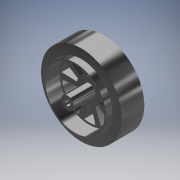
# Autodesk Inventor part: Wheel for rc car
Saved by Autodesk Inventor 2019 (Build 230136000, 136)
## iProperties
Created: 2020-03-11
Part Number: Wheel for rc car
Material: Generic
Document SubType Name: Modeling
Designer: 108863
Density: 1 g/cm^3
Appearance: Knurled 45
Author: 108863
Autodesk Inventor part; units mm, degrees
ref_plane "YZ Plane" through (0, 0, 0) normal (1, 0, 0) x (0, 1, 0)
ref_plane "XZ Plane" through (0, 0, 0) normal (0, 1, 0) x (-1, 0, 0)
sketch "Sketch2" plane through (0, 0, 0) normal (0, 0, 1) x (1, 0, 0)
  circle A0 centre (0, 0) radius 10.9728
  dimension "d5" = 21.9456
  constraints: 1 centre point, 1 coincident
  measures "d5" diameter of A0
extrude "Extrusion2" add sketch "Sketch2" along normal blind 12.4714
sketch "Sketch3" plane through (0, 0, 12.4714) normal (0, 0, 1) x (1, 0, 0)
  circle A0 centre (0, 0) radius 0.9906
  dimension "d8" = 1.9812
  constraints: 1 centre point, 1 coincident
  measures "d8" diameter of A0
extrude "Extrusion3" cut sketch "Sketch3" against normal blind 6.2484
sketch "Sketch4" plane through (0, 0, 0) normal (0, 0, -1) x (-1, 0, 0)
  circle A0 centre (0, 0) radius 4.3117
  circle A1 centre (0, 0) radius 10.9728 projected
  line L0 (-1.7142, 3.9562) -> (-3.3109, 9.1407)
  line L1 (-0.564, 4.2746) -> (-2.0134, 9.5111)
  line L2 (-0.564, 4.2746) -> (-1.7142, 3.9562)
  line L3 (0, -15.3619) -> (0, 15.3619) projected
  circle A2 centre (0, 0) radius 9.7218
  line L4 (-3.7122, 2.1931) -> (-8.0513, 5.4489)
  line L5 (-2.9688, 3.1267) -> (-7.2193, 6.5112)
  line L6 (-2.9688, 3.1267) -> (-3.7122, 2.1931)
  line L7 (-4.2923, -0.4077) -> (-9.7164, -0.3242)
  line L8 (-4.2397, 0.7845) -> (-9.6677, 1.0243)
  line L9 (-4.2397, 0.7845) -> (-4.2923, -0.4077)
  line L10 (-3.2329, -2.8528) -> (-7.6702, -5.9735)
  line L11 (-3.8911, -1.8573) -> (-8.4234, -4.8539)
  line L12 (-3.8911, -1.8573) -> (-3.2329, -2.8528)
  line L13 (-0.9386, -4.2082) -> (-2.6942, -9.3411)
  line L14 (-2.0563, -3.7897) -> (-3.9616, -8.8781)
  line L15 (-2.0563, -3.7897) -> (-0.9386, -4.2082)
  line L16 (1.7142, -3.9562) -> (3.3109, -9.1407)
  line L17 (0.564, -4.2746) -> (2.0134, -9.5111)
  line L18 (0.564, -4.2746) -> (1.7142, -3.9562)
  line L19 (3.7122, -2.1931) -> (8.0513, -5.4489)
  line L20 (2.9688, -3.1267) -> (7.2193, -6.5112)
  line L21 (2.9688, -3.1267) -> (3.7122, -2.1931)
  line L22 (4.2923, 0.4077) -> (9.7164, 0.3242)
  line L23 (4.2397, -0.7845) -> (9.6677, -1.0243)
  line L24 (4.2397, -0.7845) -> (4.2923, 0.4077)
  line L25 (3.2329, 2.8528) -> (7.6702, 5.9735)
  line L26 (3.8911, 1.8573) -> (8.4234, 4.8539)
  line L27 (3.8911, 1.8573) -> (3.2329, 2.8528)
  line L28 (0.9386, 4.2082) -> (2.6942, 9.3411)
  line L29 (2.0563, 3.7897) -> (3.9616, 8.8781)
  line L30 (2.0563, 3.7897) -> (0.9386, 4.2082)
  line L31 (-2.8801, 3.2086) -> (-7.0341, 6.7108)
  line L32 (-3.739, 8.9741) -> (-1.8992, 3.8708)
  line L33 (-2.8801, 3.2086) -> (-1.8992, 3.8708)
  dimension "d11" = 8.6233
  dimension "d12" = 19.4437
  dimension "d15" = 360
  constraints: 66 end point, 8 point on circle, 2 centre point, 2 coincident, 2 equal length, 1 perpendicular, 71 other
  measures "d11" diameter of A0
  measures "d12" diameter of A2
extrude "Extrusion4" cut sketch "Sketch4" against normal through all contours A0 L31 A2 L32
pattern_circular "Circular Pattern1" count 10 over 360 about axis through (0, 0, 0) along (0, 0, 1) of "Extrusion4"
ref_plane "Work Plane1" through (0, 0, 6.2357) normal (0, 0, -1) x (-1, 0, 0)
sketch "Sketch5" plane through (0, 0, 6.2357) normal (0, 0, -1) x (-1, 0, 0)
  arc A0 (-8.2998, 5.0625) -> (-9.6353, 1.2946) centre (0, 0) ccw projected
  arc A1 (-3.8117, 2.0153) -> (-4.216, 0.903) centre (0, 0) ccw projected
  arc A2 (-9.6903, -0.7829) -> (-8.556, -4.6161) centre (0, 0) ccw projected
  arc A3 (-4.2683, -0.6101) -> (-3.9416, -1.7476) centre (0, 0) ccw projected
  arc A4 (-7.3795, -6.3291) -> (-4.2087, -8.7636) centre (0, 0) ccw projected
  arc A5 (-3.0945, -3.0024) -> (-2.1616, -3.7307) centre (0, 0) ccw projected
  arc A6 (-2.2499, -9.4579) -> (1.7462, -9.5637) centre (0, 0) ccw projected
  arc A7 (-0.7388, -4.2479) -> (0.4441, -4.2887) centre (0, 0) ccw projected
  arc A8 (3.739, -8.9741) -> (7.0341, -6.7108) centre (0, 0) ccw projected
  arc A9 (1.8992, -3.8708) -> (2.8801, -3.2086) centre (0, 0) ccw projected
  arc A10 (8.2998, -5.0625) -> (9.6353, -1.2946) centre (0, 0) ccw projected
  arc A11 (3.8117, -2.0153) -> (4.216, -0.903) centre (0, 0) ccw projected
  arc A12 (9.6903, 0.7829) -> (8.556, 4.6161) centre (0, 0) ccw projected
  arc A13 (4.2683, 0.6101) -> (3.9416, 1.7476) centre (0, 0) ccw projected
  arc A14 (7.3795, 6.3291) -> (4.2087, 8.7636) centre (0, 0) ccw projected
  arc A15 (3.0945, 3.0024) -> (2.1616, 3.7307) centre (0, 0) ccw projected
  arc A16 (2.2499, 9.4579) -> (-1.7462, 9.5637) centre (0, 0) ccw projected
  arc A17 (0.7388, 4.2479) -> (-0.4441, 4.2887) centre (0, 0) ccw projected
  arc A18 (-1.8992, 3.8708) -> (-2.8801, 3.2086) centre (0, 0) ccw projected
  arc A19 (-3.739, 8.9741) -> (-7.0341, 6.7108) centre (0, 0) ccw projected
  circle A20 centre (0, 0) radius 10.9728 projected
  circle A21 centre (0, 0) radius 14.2367
  line L0 (-4.216, 0.903) -> (-9.6353, 1.2946) projected
  line L1 (-8.2998, 5.0625) -> (-3.8117, 2.0153) projected
  line L2 (-3.9416, -1.7476) -> (-8.556, -4.6161) projected
  line L3 (-9.6903, -0.7829) -> (-4.2683, -0.6101) projected
  line L4 (-2.1616, -3.7307) -> (-4.2087, -8.7636) projected
  line L5 (-7.3795, -6.3291) -> (-3.0945, -3.0024) projected
  line L6 (0.4441, -4.2887) -> (1.7462, -9.5637) projected
  line L7 (-2.2499, -9.4579) -> (-0.7388, -4.2479) projected
  line L8 (2.8801, -3.2086) -> (7.0341, -6.7108) projected
  line L9 (3.739, -8.9741) -> (1.8992, -3.8708) projected
  line L10 (4.216, -0.903) -> (9.6353, -1.2946) projected
  line L11 (8.2998, -5.0625) -> (3.8117, -2.0153) projected
  line L12 (3.9416, 1.7476) -> (8.556, 4.6161) projected
  line L13 (9.6903, 0.7829) -> (4.2683, 0.6101) projected
  line L14 (2.1616, 3.7307) -> (4.2087, 8.7636) projected
  line L15 (7.3795, 6.3291) -> (3.0945, 3.0024) projected
  line L16 (-0.4441, 4.2887) -> (-1.7462, 9.5637) projected
  line L17 (2.2499, 9.4579) -> (0.7388, 4.2479) projected
  line L18 (-3.739, 8.9741) -> (-1.8992, 3.8708) projected
  line L19 (-2.8801, 3.2086) -> (-7.0341, 6.7108) projected
  dimension "d23" = 3.2639
  constraints: 1 centre point, 1 coincident
  measures "d23" radial gap between concentric circles of A21 A20
extrude "Extrusion5" add sketch "Sketch5" along normal mid plane 7.9629 contours A21
sketch "Sketch8" plane through (0, 0, 12.4714) normal (0, 0, 1) x (1, 0, 0)
  circle A0 centre (0, 0) radius 10.4372
  constraints: 1 centre point, 1 coincident
extrude "Extrusion8" cut sketch "Sketch8" against normal blind 4.9784
sketch "Sketch9" plane through (0, 0, 0) normal (0, 0, -1) x (-1, 0, 0)
  line L0 (-3.6662, 0) -> (-1.8331, 3.175)
  line L1 (-1.8331, 3.175) -> (1.8331, 3.175)
  line L2 (1.8331, 3.175) -> (3.6662, 0)
  line L3 (3.6662, 0) -> (1.8331, -3.175)
  line L4 (1.8331, -3.175) -> (-1.8331, -3.175)
  line L5 (-1.8331, -3.175) -> (-3.6662, 0)
  point P0 (0, 0)
  point P1 (0, 0)
  dimension "d34" = 6.35
  constraints: 12 end point, 1 coincident, 13 other
  measures "d34" distance between parallel lines of L4 L1
extrude "Extrusion9" add sketch "Sketch9" along normal blind 0.7747
sketch "Sketch10" plane through (0, 0, 7.493) normal (0, 0, 1) x (1, 0, 0)
  circle A0 centre (0, 0) radius 2.286
  circle A1 centre (0, 0) radius 0.9906 projected
  dimension "d38" = 1.2954
  constraints: 1 centre point, 1 coincident
  measures "d38" radial gap between concentric circles of A0 A1
extrude "Extrusion10" add sketch "Sketch10" along normal blind 8
scale "Scale1" factors (2, 2, 2) then translate (0, 0, -6.2357) bodies 1
scale "Scale2" factors (2, 2, 2) then translate (0, 0, -6.2357) bodies 1
body "Solid2"
